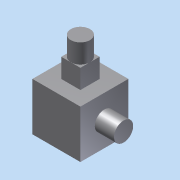
# Autodesk Inventor part: cubo 2
Saved by Autodesk Inventor 2012 (Build 160160000, 160)
## iProperties
Created: 2019-02-27
Part Number: cubo 2
Material: Default
Document SubType Name: Modeling
Designer: breno.freitas
Density: 1 g/cm^3
Author: breno.freitas
Autodesk Inventor part; units mm, degrees
ref_plane "YZ Plane" through (0, 0, 0) normal (1, 0, 0) x (0, 1, 0)
ref_plane "XZ Plane" through (0, 0, 0) normal (0, 1, 0) x (-1, 0, 0)
ref_plane "XY Plane" through (0, 0, 0) normal (0, 0, 1) x (1, 0, 0)
sketch "Sketch1" plane through (0, 0, 0) normal (0, 0, 1) x (1, 0, 0)
  line L0 (-25, 25) -> (25, 25)
  line L1 (25, 25) -> (25, -25)
  line L2 (25, -25) -> (-25, -25)
  line L3 (-25, -25) -> (-25, 25)
  point P0 (0, 0)
  point P1 (-25, 0)
  point P2 (0, 25)
  dimension "d0" = 50
  dimension "d1" = 50
  constraints: 8 end point, 2 midpoint, 2 parallel, 1 horizontal, 1 horizontal alignment, 1 perpendicular, 1 vertical alignment
  measures "d0" distance of L2.end L0.start
  measures "d1" distance of L0.start L0.end
extrude "Extrusion1" add sketch "Sketch1" against normal blind 50
sketch "Sketch2" plane through (0, 0, 0) normal (0, 0, 1) x (1, 0, 0)
  line L0 (-10, 10) -> (10, 10)
  line L1 (10, 10) -> (10, -10)
  line L2 (10, -10) -> (-10, -10)
  line L3 (-10, -10) -> (-10, 10)
  point P0 (0, 0)
  point P1 (-10, 0)
  point P2 (0, 10)
  dimension "d4" = 20
  dimension "d5" = 20
  constraints: 8 end point, 2 midpoint, 2 parallel, 1 horizontal, 1 horizontal alignment, 1 perpendicular, 1 vertical alignment
  measures "d4" distance of L0.start L0.end
  measures "d5" distance of L0.end L1.end
extrude "Extrusion2" add sketch "Sketch2" along normal blind 20
sketch "Sketch3" plane through (0, 0, 20) normal (0, 0, 1) x (1, 0, 0)
  line L0 (10, 10) -> (10, -10) projected
  circle A0 centre (0, 0) radius 10
  constraints: 1 centre point, 1 coincident, 1 tangent
extrude "Extrusion3" add sketch "Sketch3" along normal blind 20
sketch "Sketch4" plane through (25, -25, 0) normal (1, 0, 0) x (0, 0, -1)
  line L0 (50, 0) -> (50, 50) projected
  line L1 (0, 50) -> (50, 50) projected
  circle A0 centre (25, 25) radius 10
  point P0 (0, 25)
  point P1 (50, 25)
  point P2 (25, 50)
  dimension "d10" = 20
  constraints: 2 midpoint, 1 centre point, 1 horizontal alignment, 1 vertical alignment
  measures "d10" diameter of A0
extrude "Extrusion4" add sketch "Sketch4" along normal blind 20
body "Solid1"
